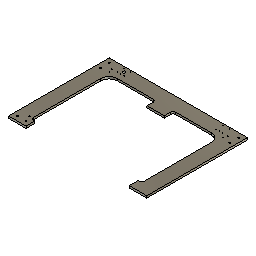
Mark3_larger_corexy (Autodesk Fusion 360 design; units mm, degrees)
Autodesk Fusion 360 part; units mm, degrees
sketch "Sketch1" plane through (0, 0, 0) normal (0, 0, 1) x (1, 0, 0)
  line L0 (315.9125, 230.1875) -> (-315.9125, 230.1875)
  line L1 (-315.9125, 230.1875) -> (-315.9125, -230.1875)
  line L2 (315.9125, -230.1875) -> (315.9125, 230.1875)
  line L3 (252.4125, 128.9187) -> (252.4125, -180.1875)
  line L4 (-253.4061, 128.9187) -> (-253.4061, -180.178)
  line L5 (-315.9125, -230.1875) -> (-252.4125, -230.1875) construction
  line L6 (252.4125, -230.1875) -> (315.9125, -230.1875) construction
  arc A0 (-215.3061, 167.0187) -> (-253.4061, 128.9187) centre (-215.3061, 128.9187) ccw
  arc A1 (252.4125, 128.9187) -> (214.3125, 167.0187) centre (214.3125, 128.9187) ccw
  line L7 (-315.9125, 230.1875) -> (-275.9125, 230.1875) construction
  line L8 (-315.9125, 150.1875) -> (-315.9125, 230.1875) construction
  line L9 (315.9125, 150.1875) -> (315.9125, 230.1875) construction
  line L10 (-315.9125, -230.1875) -> (-235.9125, -230.1875) construction
  line L11 (-235.9125, -230.1875) -> (-235.9125, -190.1875) construction
  line L12 (-315.9125, -190.1875) -> (-315.9125, -230.1875) construction
  line L13 (315.9125, -230.1875) -> (235.9125, -230.1875) construction
  line L14 (235.9125, -230.1875) -> (235.9125, -190.1875) construction
  line L15 (315.9125, -190.1875) -> (315.9125, -230.1875) construction
  line L16 (-315.9125, -230.1875) -> (-235.9125, -230.1875)
  line L17 (-235.9125, -190.1875) -> (-235.9125, -230.1875)
  line L18 (-235.9125, -190.1875) -> (-243.4188, -190.178)
  line L19 (315.9125, -230.1875) -> (235.9125, -230.1875)
  line L20 (235.9125, -190.1875) -> (235.9125, -230.1875)
  line L21 (235.9125, -190.1875) -> (242.4125, -190.1875)
  arc A2 (-253.4061, -180.178) -> (-243.4188, -190.178) centre (-243.4061, -180.178) ccw
  arc A3 (242.4125, -190.1875) -> (252.4125, -180.1875) centre (242.4125, -180.1875) ccw
  circle A4 centre (295.9125, 210.1875) radius 3.5
  circle A5 centre (295.9125, 170.1875) radius 3.5
  circle A6 centre (-295.9125, -210.1875) radius 3.5
  circle A7 centre (-255.9125, -210.1875) radius 3.5
  circle A8 centre (-295.9125, 210.1875) radius 3.5
  circle A9 centre (-295.9125, 170.1875) radius 3.5
  line L22 (-210.4125, 192.1875) -> (-241.4125, 192.1875) construction
  line L23 (-241.4125, 192.1875) -> (-241.4125, 223.1875) construction
  line L24 (-241.4125, 223.1875) -> (-210.4125, 223.1875) construction
  line L25 (-210.4125, 223.1875) -> (-210.4125, 192.1875) construction
  line L26 (241.4125, 192.1875) -> (210.4125, 192.1875) construction
  line L27 (210.4125, 192.1875) -> (210.4125, 223.1875) construction
  line L28 (210.4125, 223.1875) -> (241.4125, 223.1875) construction
  line L29 (241.4125, 223.1875) -> (241.4125, 192.1875) construction
  circle A10 centre (210.4125, 223.1875) radius 1.5
  circle A11 centre (241.4125, 223.1875) radius 1.5
  circle A12 centre (241.4125, 192.1875) radius 1.5
  circle A13 centre (210.4125, 192.1875) radius 1.5
  circle A14 centre (-241.4125, 223.1875) radius 1.5
  circle A15 centre (-210.4125, 223.1875) radius 1.5
  circle A16 centre (-210.4125, 192.1875) radius 1.5
  circle A17 centre (-241.4125, 192.1875) radius 1.5
  line L30 (-255.3025, -256.6509) -> (-267.5225, -256.6509) construction
  circle A18 centre (-265.4125, 190.6875) radius 2.1
  circle A19 centre (-259.1925, 174.9546) radius 2.1
  circle A20 centre (-225.9125, 192.1875) radius 2.1
  circle A21 centre (259.1925, 174.9546) radius 2.1
  circle A22 centre (225.9125, 192.1875) radius 2.1
  circle A23 centre (265.4125, 190.6875) radius 2.1
  line L31 (-40.4968, 157.0187) -> (-40.4968, 127.0187)
  line L32 (-40.4968, 127.0187) -> (39.5032, 127.0187)
  line L33 (39.5032, 127.0187) -> (39.5032, 157.0187)
  line L34 (-215.3061, 167.0187) -> (-50.4968, 167.0187)
  line L35 (49.5032, 167.0187) -> (214.3125, 167.0187)
  arc A24 (-40.4968, 157.0187) -> (-50.4968, 167.0187) centre (-50.4968, 157.0187) ccw
  arc A25 (49.5032, 167.0187) -> (39.5032, 157.0187) centre (49.5032, 157.0187) ccw
  circle A26 centre (-266.8549, -183.6966) radius 2.5
  circle A27 centre (-225.9125, 207.6875) radius 6.075
  line L36 (711.2, -330.2) -> (711.2, 279.4)
  line L37 (711.2, 279.4) -> (1320.8, 279.4)
  line L38 (1320.8, 279.4) -> (1320.8, -330.2)
  line L39 (791.1998, -330.2) -> (791.1998, -290.8859)
  line L40 (1257.3, -273.4361) -> (1257.3, 177.8)
  line L41 (774.7, -273.4361) -> (774.7, 177.8)
  line L42 (711.2, 279.4) -> (711.2, 215.9)
  line L43 (791.1998, -290.8859) -> (792.1498, -290.8859)
  line L44 (1240.8001, -330.2) -> (1240.8001, -290.8859)
  line L45 (1240.8001, -290.8859) -> (1239.8502, -290.8859)
  line L46 (1240.8001, -330.2) -> (1320.8, -330.2)
  line L47 (711.2, -330.2) -> (791.1998, -330.2)
  arc A28 (812.8, 215.9) -> (774.7, 177.8) centre (812.8, 177.8) ccw
  arc A29 (1257.3, 177.8) -> (1219.2, 215.9) centre (1219.2, 177.8) ccw
  arc A30 (774.7, -273.4361) -> (792.1498, -290.8859) centre (792.1498, -273.4361) ccw
  arc A31 (1239.8502, -290.8859) -> (1257.3, -273.4361) centre (1239.8502, -273.4361) ccw
  circle A32 centre (731.1999, -310.5429) radius 4
  circle A33 centre (771.1999, -310.5429) radius 4
  circle A34 centre (1260.8001, -310.5429) radius 4
  circle A35 centre (1300.8001, -310.5429) radius 4
  line L48 (1056, 175.9) -> (976, 175.9)
  line L49 (976, 175.9) -> (976, 198.4502)
  line L50 (1056, 198.4502) -> (1056, 175.9)
  line L51 (1056, 175.9) -> (976, 255.9) construction
  line L52 (976, 175.9) -> (1056, 255.9) construction
  line L53 (812.8, 215.9) -> (958.5502, 215.9)
  line L54 (1073.4498, 215.9) -> (1219.2, 215.9)
  arc A36 (1073.4498, 215.9) -> (1056, 198.4502) centre (1073.4498, 198.4502) ccw
  arc A37 (976, 198.4502) -> (958.5502, 215.9) centre (958.5502, 198.4502) ccw
  line L55 (1244.6, -286.0929) -> (787.4, -286.0929)
  line L56 (787.4, -286.0929) -> (787.4, 158.4071)
  line L57 (787.4, 158.4071) -> (1244.6, 158.4071)
  line L58 (1244.6, 158.4071) -> (1244.6, -286.0929)
  line L59 (1244.6, -286.0929) -> (787.4, 158.4071) construction
  line L60 (787.4, -286.0929) -> (1244.6, 158.4071) construction
  point P0 (-295.9125, 210.1875)
  point P1 (-295.9125, 170.1875)
  point P2 (295.9125, 210.1875)
  point P3 (295.9125, 170.1875)
  point P4 (-255.9125, -210.1875)
  point P5 (-295.9125, -210.1875)
  point P6 (295.9125, -210.1875)
  point P7 (255.9125, -210.1875)
  point P8 (-225.9125, 207.6875)
  point P9 (-225.9125, 207.6875)
  point P10 (-225.9125, 207.6875)
  point P11 (225.9125, 207.6875)
  point P12 (225.9125, 207.6875)
  point P13 (-259.1925, 174.9546)
  point P14 (259.1925, 174.9546)
  point P15 (225.9125, 192.1875)
  point P16 (265.4125, 190.6875)
  point P17 (-266.8549, -183.6966)
  point P18 (791.1998, -330.2)
  point P19 (731.1999, -310.5429)
  point P20 (771.1999, -310.5429)
  point P21 (1260.8001, -310.5429)
  point P22 (1300.8001, -310.5429)
  point P23 (1016, -63.8429)
  point P24 (1016, -63.8429)
  dimension "d1" = 460.375
  dimension "d2" = 631.825
  dimension "d6" = 38.1
  dimension "d7" = 38.1
  dimension "d8" = 40
  dimension "d9" = 80
  dimension "d10" = 80
  dimension "d12" = 80
  dimension "d13" = 40
  dimension "d14" = 80
  dimension "d15" = 40
  dimension "d16" = 10
  dimension "d17" = 10
  dimension "d19" = 40
  dimension "d23" = 40
  dimension "d24" = 7
  dimension "d25" = 7
  dimension "d27" = 40
  dimension "d28" = 7
  dimension "d29" = 7
  dimension "d31" = 40
  dimension "d34" = 7
  dimension "d35" = 7
  dimension "d38" = 31
  dimension "d39" = 31
  dimension "d43" = 31
  dimension "d44" = 31
  dimension "d45" = 3
  dimension "d46" = 3
  dimension "d47" = 3
  dimension "d48" = 3
  dimension "d49" = 3
  dimension "d50" = 3
  dimension "d51" = 3
  dimension "d52" = 3
  dimension "d67" = 12.22
  dimension "d77" = 4.2
  dimension "d78" = 4.2
  dimension "d79" = 4.2
  dimension "d82" = 4.2
  dimension "d84" = 4.2
  dimension "d87" = 4.2
  dimension "d98" = 80
  dimension "d99" = 10
  dimension "d192" = 5
  dimension "d196" = 12.15
  dimension "d217" = 609.6
  dimension "d218" = 609.6
  dimension "d219" = 79.9998
  dimension "d220" = 79.9998
  dimension "d221" = 39.3141
  dimension "d224" = 63.5
  dimension "d225" = 39.3141
  dimension "d226" = 38.1
  dimension "d227" = 38.1
  dimension "d228" = 17.4498
  dimension "d229" = 17.4498
  dimension "d242" = 8
  dimension "d243" = 8
  dimension "d246" = 8
  dimension "d247" = 8
  dimension "d248" = 80
  dimension "d249" = 80
  dimension "d250" = 17.4498
  dimension "d251" = 17.4498
  dimension "d252" = 444.5
  dimension "d253" = 457.2
  dimension "d254" = 457.2
  constraint perpendicular L0 L1
  constraint parallel L0 L5
  constraint parallel L1 L2
  constraint horizontal L0
  constraint coincident L6.start L5
  constraint perpendicular L3 L5
  constraint perpendicular L0 L4
  constraint perpendicular L2 L34
  constraint collinear L5 L6
  constraint tangent A0 L34
  constraint tangent L4 A0
  constraint tangent L3 A1
  constraint tangent A1 L34
  constraint horizontal L7
  constraint vertical L8
  constraint vertical L9
  constraint horizontal L10
  constraint vertical L11
  constraint vertical L12
  constraint horizontal L13
  constraint vertical L14
  constraint vertical L15
  constraint perpendicular L3 L21
  constraint tangent L4 A2
  constraint tangent L18 A2
  constraint tangent L3 A3
  constraint tangent L21 A3
  constraint coincident P2 A4.centre
  constraint coincident P3 A5.centre
  constraint coincident P5 A6.centre
  constraint coincident P4 A7.centre
  constraint coincident P0 A8.centre
  constraint coincident P1 A9.centre
  constraint perpendicular L22 L23
  constraint parallel L22 L24
  constraint parallel L23 L25
  constraint horizontal L22
  constraint coincident P10 P9
  constraint perpendicular L26 L27
  constraint parallel L26 L28
  constraint parallel L27 L29
  constraint horizontal L26
  constraint coincident P12 P11
  constraint coincident L27.end L28.start
  constraint coincident L28.end L29.start
  constraint coincident L26.start L29.end
  constraint coincident L26.end L27.start
  constraint coincident L23.end L24.start
  constraint coincident L24.end L25.start
  constraint coincident L22.start L25.end
  constraint coincident L22.end L23.start
  constraint coincident P14 A21.centre
  constraint midpoint L26 P15
  constraint collinear L34 L35
  constraint tangent L31 A24
  constraint tangent L34 A24
  constraint tangent L33 A25
  constraint tangent L35 A25
  constraint equal A24 A25
  constraint coincident P17 A26.centre
  constraint parallel L36 L38
  constraint coincident P18 L39.start
  constraint perpendicular L37 L40
  constraint perpendicular L37 L41
  constraint perpendicular L37 L42
  constraint perpendicular L38 L53
  constraint perpendicular L39 L43
  constraint perpendicular L38 L45
  constraint perpendicular L38 L46
  constraint perpendicular L39 L47
  constraint tangent L41 A28
  constraint tangent A28 L53
  constraint tangent L40 A29
  constraint tangent A29 L53
  constraint tangent L43 A30
  constraint tangent L41 A30
  constraint tangent L45 A31
  constraint tangent L40 A31
  constraint coincident P19 A32.centre
  constraint coincident P20 A33.centre
  constraint coincident P21 A34.centre
  constraint coincident P22 A35.centre
  constraint perpendicular L48 L49
  constraint parallel L49 L50
  constraint horizontal L48
  constraint collinear L53 L54
  constraint tangent L50 A36
  constraint tangent L54 A36
  constraint tangent L49 A37
  constraint tangent L53 A37
  constraint perpendicular L55 L56
  constraint parallel L55 L57
  constraint parallel L56 L58
  constraint horizontal L55
  constraint coincident L59 P24
  constraint coincident L60 P24
  constraint coincident P24 P23
  measures "d1" distance of L0.end L1.end
  measures "d2" distance of L1.end L2.start
  measures "d6" radius of A0
  measures "d7" radius of A1
  measures "d8" distance of L0.end L7.end
  measures "d9" distance of L0.end L8.start
  measures "d10" distance of L0.start L9.start
  measures "d12" distance of L1.end L10.end
  measures "d13" distance of L1.end L12.start
  measures "d14" distance of L2.start L13.end
  measures "d15" distance of L2.start L15.start
  measures "d16" radius of A2
  measures "d17" radius of A3
  measures "d19" distance of P0 P1
  measures "d23" distance of P2 P3
  measures "d24" diameter of A4
  measures "d25" diameter of A5
  measures "d27" distance of P4 P5
  measures "d28" diameter of A6
  measures "d29" diameter of A7
  measures "d31" distance of P6 P7
  measures "d34" diameter of A8
  measures "d35" diameter of A9
  measures "d38" distance of L22.end L23.end
  measures "d39" distance of L23.end L24.end
  measures "d43" distance of L26.end L27.end
  measures "d44" distance of L27.end L28.end
  measures "d45" diameter of A10
  measures "d46" diameter of A11
  measures "d47" diameter of A12
  measures "d48" diameter of A13
  measures "d49" diameter of A14
  measures "d50" diameter of A15
  measures "d51" diameter of A16
  measures "d52" diameter of A17
  measures "d67" distance of L30.start L30.end
  measures "d77" diameter of A18
  measures "d78" diameter of A19
  measures "d79" diameter of A20
  measures "d82" diameter of A21
  measures "d84" diameter of A22
  measures "d87" diameter of A23
  measures "d98" distance of L31.end L32.end
  measures "d99" radius of A24
  measures "d192" diameter of A26
  measures "d196" diameter of A27
  measures "d217" distance of L36.end L37.end
  measures "d218" distance of L36.start L36.end
  measures "d219" distance of L36.start P18
  measures "d220" distance of L38.end L44.start
  measures "d221" distance of P18 L39.end
  measures "d224" distance of L36.end L42.end
  measures "d225" distance of L44.start L44.end
  measures "d226" radius of A28
  measures "d227" radius of A29
  measures "d228" radius of A30
  measures "d229" radius of A31
  measures "d242" diameter of A32
  measures "d243" diameter of A33
  measures "d246" diameter of A34
  measures "d247" diameter of A35
  measures "d248" distance of L51.end L52.end
  measures "d249" distance of L48.end L51.end
  measures "d250" radius of A36
  measures "d251" radius of A37
  measures "d252" distance of L55.end L56.end
  measures "d253" distance of L56.end L57.end
  measures "d254" distance of L55.start L55.end
sketch "Sketch2" plane through (0, 0, 0) normal (0, 0, 1) x (1, 0, 0)
sketch "Sketch3" plane through (0, 0, 9.906) normal (0, 0, 1) x (-1, 0, 0)
  circle A0 centre (259.1925, -174.9546) radius 2.1
  circle A1 centre (225.9125, -192.1875) radius 2.1
  circle A2 centre (-259.1925, -174.9546) radius 2.1
  circle A3 centre (-225.9125, -192.1875) radius 2.1
  circle A4 centre (-265.4125, -190.6875) radius 2.1
  circle A5 centre (-210.4125, -223.1875) radius 1.5
  circle A6 centre (-241.4125, -223.1875) radius 1.5
  circle A7 centre (241.4125, -223.1875) radius 1.5
  circle A8 centre (210.4125, -223.1875) radius 1.5
  circle A9 centre (210.4125, -192.1875) radius 1.5
  circle A10 centre (241.4125, -192.1875) radius 1.5
  circle A11 centre (265.4125, -190.6875) radius 2.1
  circle A12 centre (295.9125, -170.1875) radius 3.5
  circle A13 centre (295.9125, -210.1875) radius 3.5
  circle A14 centre (255.9125, 210.1875) radius 3.5
  circle A15 centre (295.9125, 210.1875) radius 3.5
  circle A16 centre (-295.9125, -170.1875) radius 3.5
  circle A17 centre (-295.9125, -210.1875) radius 3.5
  circle A18 centre (-241.4125, -192.1875) radius 1.5
  circle A19 centre (-210.4125, -192.1875) radius 1.5
  line L0 (-235.9125, 190.1875) -> (-235.9125, 230.1875)
  line L1 (-235.9125, 230.1875) -> (-315.9125, 230.1875)
  line L2 (-315.9125, 230.1875) -> (-315.9125, -230.1875)
  line L3 (-315.9125, -230.1875) -> (315.9125, -230.1875)
  line L4 (315.9125, -230.1875) -> (315.9125, 230.1875)
  line L5 (315.9125, 230.1875) -> (235.9125, 230.1875)
  line L6 (235.9125, 230.1875) -> (235.9125, 190.1875)
  line L7 (235.9125, 190.1875) -> (243.4188, 190.178)
  arc A20 (253.4061, 180.178) -> (243.4188, 190.178) centre (243.4061, 180.178) ccw
  line L8 (253.4061, 180.178) -> (253.4061, -128.9187)
  arc A21 (215.3061, -167.0187) -> (253.4061, -128.9187) centre (215.3061, -128.9187) ccw
  line L9 (215.3061, -167.0187) -> (50.4968, -167.0187)
  arc A22 (-252.4125, -128.9187) -> (-214.3125, -167.0187) centre (-214.3125, -128.9187) ccw
  arc A23 (-242.4125, 190.1875) -> (-252.4125, 180.1875) centre (-242.4125, 180.1875) ccw
  line L10 (-242.4125, 190.1875) -> (-235.9125, 190.1875)
  circle A24 centre (-225.9125, -207.6875) radius 6.075
  circle A25 centre (-266.8549, 183.6966) radius 2.5
  circle A26 centre (20.4968, -147.0187) radius 3.5
  circle A27 centre (-19.5032, -147.0187) radius 3.5
  circle A28 centre (-296.8977, -139.8125) radius 1.5
  circle A29 centre (-296.8977, -89.8125) radius 1.5
  circle A30 centre (-296.8977, -39.8125) radius 1.5
  circle A31 centre (-296.8977, 10.1875) radius 1.5
  circle A32 centre (-296.8977, 60.1875) radius 1.5
  circle A33 centre (-296.8977, 110.1875) radius 1.5
  circle A34 centre (-296.8977, 160.1875) radius 1.5
  circle A35 centre (-295.9125, 210.1875) radius 3.5
  circle A36 centre (-255.9125, 210.1875) radius 3.5
  circle A37 centre (296.8977, 165.5641) radius 1.5
  circle A38 centre (296.8977, 115.5641) radius 1.5
  circle A39 centre (296.8977, 60.1875) radius 1.5
  circle A40 centre (296.8977, 10.1875) radius 1.5
  circle A41 centre (296.8977, -39.8125) radius 1.5
  circle A42 centre (296.8977, -89.8125) radius 1.5
  circle A43 centre (296.8977, -139.8125) radius 1.5
  point P0 (-266.8549, 183.6966)
  point P1 (296.8977, -139.8125)
  point P2 (20.4968, -147.0187)
  point P3 (-19.5032, -147.0187)
  point P4 (-295.9125, 210.1875)
  point P5 (-295.9125, 210.1875)
  point P6 (-255.9125, 210.1875)
  point P7 (-255.9125, 210.1875)
  point P8 (-242.0032, -117.0187)
  point P9 (-242.0032, 182.9813)
  point P10 (242.9968, 182.9813)
  point P11 (242.9968, -117.0187)
  point P12 (296.8977, -89.8125)
  point P13 (296.8977, -39.8125)
  point P14 (296.8977, 10.1875)
  point P15 (296.8977, 115.5641)
  point P16 (296.8977, 60.1875)
  point P17 (296.8977, 165.5641)
  point P18 (-296.8977, -139.8125)
  point P19 (-296.8977, -89.8125)
  point P20 (-296.8977, -39.8125)
  point P21 (-296.8977, 10.1875)
  point P22 (-296.8977, 60.1875)
  point P23 (-296.8977, 110.1875)
  point P24 (-296.8977, 160.1875)
  point P25 (-225.9125, -207.6875)
  point P26 (-254.6349, 11.7418)
  dimension "d137" = 485
  dimension "d139" = 485
  dimension "d140" = 50
  dimension "d141" = 50
  dimension "d144" = 55.3766
  dimension "d145" = 50
  dimension "d162" = 50
  dimension "d163" = 50
  dimension "d164" = 50
  dimension "d165" = 50
  dimension "d166" = 50
  dimension "d167" = 50
  dimension "d174" = 12.15
  dimension "d193" = 5
  dimension "d194" = 7
  dimension "d195" = 7
  dimension "d197" = 3
  dimension "d198" = 3
  dimension "d199" = 3
  dimension "d200" = 3
  dimension "d201" = 3
  dimension "d202" = 3
  dimension "d203" = 3
  dimension "d204" = 7
  dimension "d205" = 7
  dimension "d206" = 3
  dimension "d207" = 3
  dimension "d208" = 3
  dimension "d209" = 3
  dimension "d210" = 3
  dimension "d211" = 3
  dimension "d212" = 3
  constraint coincident P5 P4
  constraint coincident P7 P6
  constraint coincident P25 A24.centre
  constraint coincident P0 A25.centre
  constraint coincident P2 A26.centre
  constraint coincident P3 A27.centre
  constraint coincident P18 A28.centre
  constraint coincident P19 A29.centre
  constraint coincident P20 A30.centre
  constraint coincident P21 A31.centre
  constraint coincident P22 A32.centre
  constraint coincident P23 A33.centre
  constraint coincident P24 A34.centre
  constraint coincident P17 A37.centre
  constraint coincident P15 A38.centre
  constraint coincident P16 A39.centre
  constraint coincident P14 A40.centre
  constraint coincident P13 A41.centre
  constraint coincident P12 A42.centre
  constraint coincident P1 A43.centre
  measures "d137" distance of P8 P11
  measures "d139" distance of P9 P10
  measures "d140" distance of P1 P12
  measures "d141" distance of P12 P13
  measures "d144" distance of P15 P16
  measures "d145" distance of P15 P17
  measures "d162" distance of P18 P19
  measures "d163" distance of P19 P20
  measures "d164" distance of P20 P21
  measures "d165" distance of P21 P22
  measures "d166" distance of P22 P23
  measures "d167" distance of P23 P24
  measures "d174" diameter of A24
  measures "d193" diameter of A25
  measures "d194" diameter of A26
  measures "d195" diameter of A27
  measures "d197" diameter of A28
  measures "d198" diameter of A29
  measures "d199" diameter of A30
  measures "d200" diameter of A31
  measures "d201" diameter of A32
  measures "d202" diameter of A33
  measures "d203" diameter of A34
  measures "d204" diameter of A35
  measures "d205" diameter of A36
  measures "d206" diameter of A37
  measures "d207" diameter of A38
  measures "d208" diameter of A39
  measures "d209" diameter of A40
  measures "d210" diameter of A41
  measures "d211" diameter of A42
  measures "d212" diameter of A43
sketch "Sketch5" plane through (0, 0, 0) normal (0, 0, 1) x (1, 0, 0)
  point P0 (-266.85, -183.7)
extrude "Extrude3" add sketch "Sketch1" along normal blind 9.525 contours L0 L1 L2 L3 L4 A0 A1 L16 L17 L18 L19 L20 L21 A2 A3 L31 L32 L33 L34 L35 A24 A25
sketch "Sketch6" plane through (0, 0, 9.525) normal (0, 0, 1) x (-1, 0, 0)
  circle A0 centre (-265.4125, -190.6875) radius 2.1
  circle A1 centre (-225.9125, -192.1875) radius 2.1
  circle A2 centre (-259.1925, -174.9546) radius 2.1
  circle A3 centre (225.9125, -192.1875) radius 2.1
  circle A4 centre (259.1925, -174.9546) radius 2.1
  circle A5 centre (265.4125, -190.6875) radius 2.1
  circle A6 centre (241.4125, -192.1875) radius 1.5
  circle A7 centre (210.4125, -192.1875) radius 1.5
  circle A8 centre (210.4125, -223.1875) radius 1.5
  circle A9 centre (241.4125, -223.1875) radius 1.5
  circle A10 centre (-210.4125, -192.1875) radius 1.5
  circle A11 centre (-241.4125, -192.1875) radius 1.5
  circle A12 centre (225.9125, -207.6875) radius 6.075
  circle A13 centre (-241.4125, -223.1875) radius 1.5
  circle A14 centre (266.8549, 183.6966) radius 2.5
  circle A15 centre (-210.4125, -223.1875) radius 1.5
  circle A16 centre (295.9125, -170.1875) radius 3.5
  circle A17 centre (295.9125, -210.1875) radius 3.5
  circle A18 centre (255.9125, 210.1875) radius 3.5
  circle A19 centre (295.9125, 210.1875) radius 3.5
  circle A20 centre (-295.9125, -170.1875) radius 3.5
  circle A21 centre (-295.9125, -210.1875) radius 3.5
  line L0 (-252.4125, -128.9187) -> (-252.4125, 180.1875)
  arc A22 (-242.4125, 190.1875) -> (-252.4125, 180.1875) centre (-242.4125, 180.1875) ccw
  line L1 (-242.4125, 190.1875) -> (-235.9125, 190.1875)
  line L2 (-235.9125, 190.1875) -> (-235.9125, 230.1875)
  line L3 (-235.9125, 230.1875) -> (-315.9125, 230.1875)
  line L4 (-315.9125, 230.1875) -> (-315.9125, -230.1875)
  line L5 (-315.9125, -230.1875) -> (315.9125, -230.1875)
  line L6 (315.9125, -230.1875) -> (315.9125, 230.1875)
  line L7 (315.9125, 230.1875) -> (235.9125, 230.1875)
  line L8 (235.9125, 230.1875) -> (235.9125, 190.1875)
  line L9 (235.9125, 190.1875) -> (243.4188, 190.178)
  arc A23 (253.4061, 180.178) -> (243.4188, 190.178) centre (243.4061, 180.178) ccw
  line L10 (253.4061, 180.178) -> (253.4061, -128.9187)
  arc A24 (215.3061, -167.0187) -> (253.4061, -128.9187) centre (215.3061, -128.9187) ccw
  line L11 (215.3061, -167.0187) -> (50.4968, -167.0187)
  arc A25 (40.4968, -157.0187) -> (50.4968, -167.0187) centre (50.4968, -157.0187) ccw
  line L12 (40.4968, -157.0187) -> (40.4968, -127.0187)
  line L13 (40.4968, -127.0187) -> (-39.5032, -127.0187)
  line L14 (-39.5032, -127.0187) -> (-39.5032, -157.0187)
  arc A26 (-49.5032, -167.0187) -> (-39.5032, -157.0187) centre (-49.5032, -157.0187) ccw
  line L15 (-49.5032, -167.0187) -> (-214.3125, -167.0187)
  arc A27 (-252.4125, -128.9187) -> (-214.3125, -167.0187) centre (-214.3125, -128.9187) ccw
  line L16 (-295.9125, -210.1875) -> (-295.9125, -230.1875)
  line L17 (-295.9125, -210.1875) -> (-315.9125, -210.1875)
  circle A28 centre (-731.1999, -259.4) radius 4
  circle A29 centre (-731.1999, -219.4) radius 4
  circle A30 centre (-1300.8, -259.4) radius 4
  circle A31 centre (-1300.8, -219.4) radius 4
  point P0 (-731.1999, -259.4)
  point P1 (-1300.8, -259.4)
  point P2 (-731.1999, -219.4)
  point P3 (-1300.8, -219.4)
  dimension "d233" = 40
  dimension "d234" = 40
  dimension "d235" = 8
  dimension "d236" = 8
  dimension "d237" = 8
  dimension "d238" = 8
  constraint coincident A21.centre L16.start
  constraint coincident L5 L16.end
  constraint perpendicular L5 L16
  constraint coincident L4 L17.end
  constraint perpendicular L4 L17
  constraint coincident P0 A28.centre
  constraint coincident P2 A29.centre
  constraint coincident P1 A30.centre
  constraint coincident P3 A31.centre
  measures "d233" distance of P0 P2
  measures "d234" distance of P1 P3
  measures "d235" diameter of A28
  measures "d236" diameter of A29
  measures "d237" diameter of A30
  measures "d238" diameter of A31
sketch "Sketch4" plane through (0, 0, 9.906) normal (0, 0, 1) x (-1, 0, 0)
  circle A0 centre (-255.9125, 210.1875) radius 3.5
  circle A1 centre (-295.9125, 210.1875) radius 3.5
  circle A2 centre (-19.5032, -147.0187) radius 3.5
  circle A3 centre (20.4968, -147.0187) radius 3.5
  circle A4 centre (-296.8977, -59.8125) radius 1.4
  circle A5 centre (-296.8977, 100.1875) radius 1.4
  circle A6 centre (296.8977, -139.8125) radius 1.4
  circle A7 centre (296.8977, 20.1875) radius 1.4
  circle A8 centre (296.8977, 180.1875) radius 1.4
  circle A9 centre (296.8977, 100.1875) radius 1.4
  circle A10 centre (296.8977, -59.8125) radius 1.4
  circle A11 centre (-296.8977, 180.1875) radius 1.4
  circle A12 centre (-296.8977, 20.1875) radius 1.4
  circle A13 centre (-296.8977, -139.8125) radius 1.4
  circle A14 centre (-266.8549, 183.6966) radius 2.1
  circle A15 centre (295.9125, 210.1875) radius 3.5
  circle A16 centre (-225.9125, -192.1875) radius 2.1
  circle A17 centre (295.9125, -210.1875) radius 3.5
  circle A18 centre (295.9125, -170.1875) radius 3.5
  circle A19 centre (255.9125, 210.1875) radius 3.5
  circle A20 centre (-295.9125, -170.1875) radius 3.5
  circle A21 centre (241.4125, -223.1875) radius 1.5
  circle A22 centre (-210.4125, -223.1875) radius 1.5
  circle A23 centre (241.4125, -192.1875) radius 1.5
  circle A24 centre (-259.1925, -174.9546) radius 2.1
  circle A25 centre (210.4125, -223.1875) radius 1.5
  circle A26 centre (259.1925, -174.9546) radius 2.1
  circle A27 centre (265.4125, -190.6875) radius 2.1
  circle A28 centre (225.9125, -192.1875) radius 2.1
  circle A29 centre (-241.4125, -223.1875) radius 1.5
  circle A30 centre (-210.4125, -192.1875) radius 1.5
  circle A31 centre (-265.4125, -190.6875) radius 2.1
  circle A32 centre (-241.4125, -192.1875) radius 1.5
  circle A33 centre (210.4125, -192.1875) radius 1.5
  circle A34 centre (-295.9125, -210.1875) radius 3.5
  circle A35 centre (265.4125, 183.6966) radius 2.1
  line L0 (-252.4125, -128.9187) -> (-252.4125, 180.1875)
  arc A36 (-242.4125, 190.1875) -> (-252.4125, 180.1875) centre (-242.4125, 180.1875) ccw
  line L1 (-242.4125, 190.1875) -> (-235.9125, 190.1875)
  line L2 (-235.9125, 190.1875) -> (-235.9125, 230.1875)
  line L3 (-235.9125, 230.1875) -> (-315.9125, 230.1875)
  line L4 (-315.9125, 230.1875) -> (-315.9125, -230.1875)
  line L5 (-315.9125, -230.1875) -> (315.9125, -230.1875)
  line L6 (315.9125, -230.1875) -> (315.9125, 230.1875)
  line L7 (315.9125, 230.1875) -> (235.9125, 230.1875)
  line L8 (235.9125, 230.1875) -> (235.9125, 190.1875)
  line L9 (235.9125, 190.1875) -> (243.4188, 190.178)
  arc A37 (253.4061, 180.178) -> (243.4188, 190.178) centre (243.4061, 180.178) ccw
  line L10 (253.4061, 180.178) -> (253.4061, -128.9187)
  arc A38 (215.3061, -167.0187) -> (253.4061, -128.9187) centre (215.3061, -128.9187) ccw
  line L11 (215.3061, -167.0187) -> (50.4968, -167.0187)
  arc A39 (40.4968, -157.0187) -> (50.4968, -167.0187) centre (50.4968, -157.0187) ccw
  line L12 (40.4968, -157.0187) -> (40.4968, -127.0187)
  line L13 (40.4968, -127.0187) -> (-39.5032, -127.0187)
  line L14 (-39.5032, -127.0187) -> (-39.5032, -157.0187)
  arc A40 (-49.5032, -167.0187) -> (-39.5032, -157.0187) centre (-49.5032, -157.0187) ccw
  line L15 (-49.5032, -167.0187) -> (-214.3125, -167.0187)
  arc A41 (-252.4125, -128.9187) -> (-214.3125, -167.0187) centre (-214.3125, -128.9187) ccw
